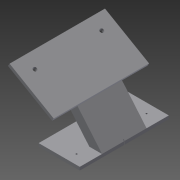
# Autodesk Inventor part: Problem Solving
Saved by Autodesk Inventor 2013 SP1 (Build 170176100, 176)
## iProperties
Created: 2013-04-06
Part Number: Problem Solving
Material: Generic
Document SubType Name: Modeling
Designer: tyler.camp
Density: 1 g/cm^3
Author: tyler.camp
Autodesk Inventor part; units mm, degrees
ref_plane "YZ Plane" through (0, 0, 0) normal (1, 0, 0) x (0, 1, 0)
ref_plane "XZ Plane" through (0, 0, 0) normal (0, 1, 0) x (-1, 0, 0)
ref_plane "XY Plane" through (0, 0, 0) normal (0, 0, 1) x (1, 0, 0)
sketch "Sketch1" plane through (0, 0, 0) normal (0, 0, 1) x (1, 0, 0)
  line L0 (28.2901, 18.0136) -> (77.2705, -40.359)
  line L1 (77.2705, -40.359) -> (51.8705, -40.359)
  line L2 (51.8705, -40.359) -> (-20.9781, 46.4586)
  line L3 (-20.9781, 46.4586) -> (28.2901, 18.0136)
  point P0 (0, 0)
  point P1 (3.656, 32.2361)
  dimension "d0" = 76.2
  dimension "d2" = 25.4
  dimension "d34" = 130
  dimension "d35" = 160
  constraints: 8 end point, 1 horizontal, 1 midpoint, 1 parallel
  measures "d0" distance of L0.start L0.end
  measures "d2" distance of L0.end L1.end
  measures "d34" angle of L1 L2
  measures "d35" angle of L0 L3
extrude "Extrusion1" add sketch "Sketch1" along normal blind 88.9
sketch "Sketch2" plane through (-20.9781, 46.4586, 0) normal (0.5, 0.8660254, 0) x (0, 0, 1)
  line L0 (0, 0) -> (0, 56.89) projected
  line L1 (-50.8, 56.89) -> (139.7, 56.89)
  line L2 (139.7, 56.89) -> (139.7, -44.71)
  line L3 (139.7, -44.71) -> (-50.8, -44.71)
  line L4 (-50.8, -44.71) -> (-50.8, 56.89)
  line L5 (0, 56.89) -> (88.9, 56.89) projected
  point P0 (0, 41.3969)
  point P1 (44.45, 19.4575)
  dimension "d6" = 190.5
  dimension "d8" = 95.25
  dimension "d9" = 101.6
  dimension "d10" = 44.45
  dimension "d11" = 88.9
  dimension "d12" = 56.89
  dimension "d45" = 0
  constraints: 8 end point, 2 parallel, 1 horizontal, 1 perpendicular
  measures "d6" distance of L1.start L1.end
  measures "d8" distance from line of L2 point (44.45, 19.458)
  measures "d9" distance of L1.end L2.end
  measures "d10" distance from line of L0 point (44.45, 19.458)
  measures "d11" distance of L0.end L5.end
  measures "d12" distance of L0.start L0.end
  measures "d45" distance between parallel lines of L5 L1
extrude "Extrusion2" add sketch "Sketch2" along normal blind 6.35
sketch "Sketch3" plane through (-17.8031, 51.9578, 0) normal (0.5, 0.8660254, 0) x (0, 0, 1)
  line L0 (139.7, 56.89) -> (-50.8, 56.89) projected
  circle A0 centre (-22.225, -19.05) radius 3.81
  circle A1 centre (111.125, -19.05) radius 3.81
  line L1 (-50.8, -44.71) -> (139.7, -44.71) projected
  line L2 (44.45, -44.71) -> (44.45, 56.89)
  line L3 (0, 0) -> (88.9, 0) projected
  point P0 (0, 41.3969)
  dimension "d17" = 7.62
  dimension "d18" = 7.62
  dimension "d19" = 0
  dimension "d46" = 133.35
  dimension "d47" = 66.675
  dimension "d86" = 19.05
  constraints: 2 centre point, 2 end point, 2 midpoint
  measures "d17" diameter of A0
  measures "d18" diameter of A1
  measures "d19" vertical distance of A1.centre A0.centre
  measures "d46" distance of A1.centre A0.centre
  measures "d47" distance from line of L2 A0.centre
  measures "d86" distance from line of A0.centre L3
extrude "Extrusion3" cut sketch "Sketch3" against normal up to next
sketch "Sketch6" plane through (-17.8031, 51.9578, 0) normal (0.5, 0.8660254, 0) x (0.8660254, -0.5, 0)
  circle A0 centre (-19.05, 22.225) radius 3.81 projected
  circle A1 centre (-19.05, -111.125) radius 3.81 projected
  line L0 (6.35, 34.925) -> (-44.45, 34.925)
  line L1 (-44.45, 34.925) -> (-44.45, -15.875)
  line L2 (-44.45, -15.875) -> (6.35, -15.875)
  line L3 (6.35, -15.875) -> (6.35, 34.925)
  line L4 (6.35, -73.025) -> (-44.45, -73.025)
  line L5 (-44.45, -73.025) -> (-44.45, -123.825)
  line L6 (-44.45, -123.825) -> (6.35, -123.825)
  line L7 (6.35, -123.825) -> (6.35, -73.025)
  point P0 (41.3969, 0)
  dimension "d52" = 50.8
  dimension "d60" = 25.4
  dimension "d61" = 25.4
  dimension "d62" = 50.8
  dimension "d63" = 12.7
  dimension "d64" = 12.7
  constraints: 16 end point, 4 parallel, 2 equal length, 2 horizontal, 2 perpendicular
  measures "d52" distance of L2.end L0.start
  measures "d60" distance from line of A0.centre L1
  measures "d61" distance from line of A1.centre L5
  measures "d62" distance of L1.end L2.end
  measures "d63" distance from line of L0 A0.centre
  measures "d64" distance from line of L6 A1.centre
extrude "Extrusion5" [suppressed]
sketch "Sketch7" plane through (-18.1206, 51.4079, 0) normal (0.5, 0.8660254, 0) x (0.8660254, -0.5, 0)
  line L0 (6.35, 38.1) -> (-44.45, 38.1) projected
  line L1 (6.35, -76.2) -> (-44.45, -76.2) projected
  line L2 (-44.45, -76.2) -> (-44.45, -127) projected
  line L3 (-44.45, -127) -> (6.35, -127) projected
  line L4 (6.35, -127) -> (6.35, -76.2) projected
  line L5 (-44.45, -12.7) -> (-39.2324, -12.7)
  line L6 (-39.2324, -12.7) -> (-39.2324, 38.1)
  line L7 (-39.2324, 38.1) -> (-44.45, 38.1)
  line L8 (-44.45, 38.1) -> (-44.45, -12.7)
  line L9 (-44.45, -127) -> (-39.2324, -127)
  line L10 (-39.2324, -127) -> (-39.2324, -76.2)
  line L11 (-39.2324, -76.2) -> (-44.45, -76.2)
  line L12 (-44.45, -76.2) -> (-44.45, -127)
  point P0 (41.3969, 0)
  dimension "d56" = 5.2176
  dimension "d57" = 5.2176
  constraints: 16 end point, 4 parallel, 2 horizontal, 2 perpendicular, 2 point on line
  measures "d56" distance between parallel lines of L8 L6
  measures "d57" distance between parallel lines of L10 L2
extrude "Extrusion6" [suppressed]
sketch "Sketch13" plane through (-57.8855, 71.4332, -38.1) normal (-0.8660254, 0.5, 0) x (0, 0, 1)
  line L0 (0, 0) -> (0, 2.54) projected
  circle A0 centre (25.4, 39.096) radius 3.175
  circle A1 centre (139.7, 39.096) radius 3.175
  line L1 (114.3, 0) -> (114.3, 2.54) projected
  point P0 (50.8, 53.34)
  point P1 (0, 53.34)
  point P2 (38.1, -32.9202)
  point P3 (114.3, 53.34)
  dimension "d98" = 6.35
  dimension "d99" = 0
  dimension "d100" = 25.4
  dimension "d101" = 50.8
  dimension "d102" = 25.4
  constraints: 2 centre point, 1 equal radius
  measures "d98" diameter of A0
  measures "d99" vertical distance of A1.centre A0.centre
  measures "d100" distance from line of L0 A0.centre
  measures "d101" distance of point (0, 53.34) point (50.8, 53.34)
  measures "d102" distance from line of L1 A1.centre
extrude "Extrusion11" [suppressed]
sketch "Sketch14" plane through (-57.8855, 71.4332, -38.1) normal (-0.8660254, 0.5, 0) x (0, 0, 1)
  circle A0 centre (25.4, 39.096) radius 3.175 projected
  line L0 (-107.95, 213.721) -> (273.05, 213.721)
  line L1 (273.05, 213.721) -> (273.05, -14.879)
  line L2 (273.05, -14.879) -> (-107.95, -14.879)
  line L3 (-107.95, -14.879) -> (-107.95, 213.721)
  point P0 (38.1, -32.9202)
  dimension "d107" = 381
  dimension "d109" = 228.6
  dimension "d110" = 133.35
  dimension "d111" = 53.975
  constraints: 8 end point, 2 parallel, 1 horizontal, 1 perpendicular
  measures "d107" distance of L0.start L0.end
  measures "d109" distance of L2.end L0.start
  measures "d110" distance from line of A0.centre L3
  measures "d111" distance from line of L2 A0.centre
extrude "Extrusion12" [suppressed]
sketch "Sketch18" plane through (-57.8855, 71.4332, -38.1) normal (0.8660254, -0.5, 0) x (0, 0, -1)
  line L0 (-273.05, -14.879) -> (107.95, -14.879) projected
  line L1 (-273.05, 213.721) -> (-195.9898, 213.721)
  line L2 (-195.9898, 213.721) -> (-195.9898, -14.879)
  line L3 (-195.9898, -14.879) -> (-273.05, -14.879)
  line L4 (-273.05, -14.879) -> (-273.05, 213.721)
  line L5 (107.95, 213.721) -> (30.8898, 213.721)
  line L6 (30.8898, 213.721) -> (30.8898, -14.879)
  line L7 (30.8898, -14.879) -> (107.95, -14.879)
  line L8 (107.95, -14.879) -> (107.95, 213.721)
  point P0 (-38.1, -32.9202)
  constraints: 16 end point, 4 parallel, 2 horizontal, 2 perpendicular, 2 point on line, 1 collinear
extrude "Extrusion14" [suppressed]
sketch "Sketch15" plane through (0, 0, 0) normal (0, 0, 1) x (1, 0, 0)
  line L0 (15.9795, 275.571) -> (4.9809, 281.921) projected
  line L1 (-109.3191, 83.9476) -> (4.9809, 281.921) projected
  line L2 (-98.3205, 77.5976) -> (-109.3191, 83.9476) projected
  line L3 (77.2705, -40.359) -> (28.2901, 18.0136) projected
  line L4 (28.2901, 18.0136) -> (-20.9781, 46.4586) projected
  line L5 (-20.9781, 46.4586) -> (51.8705, -40.359) projected
  line L6 (51.8705, -40.359) -> (77.2705, -40.359) projected
  line L7 (77.2705, -40.359) -> (-405.3295, -40.359)
  line L8 (77.2705, -40.359) -> (204.2705, -40.359)
  line L9 (-98.3205, 77.5976) -> (15.9795, 275.571) projected
  point P0 (0, 0)
  point P1 (-65.325, 58.5476)
  point P2 (48.975, 256.521)
  dimension "d125" = 127
  dimension "d127" = 482.6
  constraints: 4 end point, 3 coincident, 2 collinear
  measures "d125" distance of L7.start L8.end
  measures "d127" distance of L7.start L7.end
sketch "Sketch16" plane through (0, 0, 0) normal (0, 0, 1) x (1, 0, 0)
  line L0 (77.2705, -40.359) -> (-405.3295, -40.359) projected
  line L1 (15.9795, 275.571) -> (4.9809, 281.921) projected
  line L2 (-109.3191, 83.9476) -> (4.9809, 281.921) projected
  line L3 (-98.3205, 77.5976) -> (-109.3191, 83.9476) projected
  line L4 (77.2705, -40.359) -> (204.2705, -40.359) projected
  line L5 (-98.3205, 77.5976) -> (15.9795, 275.571) projected
  point P0 (0, 0)
  point P1 (-65.325, 58.5476)
  point P2 (51.8705, -40.359)
  point P3 (51.8705, -40.359)
  dimension "d129" = 457.2
  dimension "d130" = 322.28
  dimension "d131" = 98.9066
  dimension "d150" = 188.291
  measures "d129" distance of L0.end point (51.87, -40.359)
  measures "d130" distance from line of L4 point (4.981, 281.921)
  measures "d131" distance from line of L0 point (-65.325, 58.548)
  measures "d150" horizontal distance of L4.end L1.start
sketch "Sketch17" plane through (0, 0, 0) normal (0, 0, 1) x (1, 0, 0)
  line L0 (77.2705, -40.359) -> (-405.3295, -40.359) projected
  line L1 (-144.0325, 61.241) -> (-144.0325, -40.359)
  line L2 (-144.0325, -40.359) -> (-42.4325, -40.359)
  line L3 (-42.4325, -40.359) -> (-42.4325, 35.841)
  line L4 (-42.4325, 35.841) -> (-144.0325, 61.241)
  line L5 (77.2705, -40.359) -> (204.2705, -40.359) projected
  point P0 (0, 0)
  point P1 (-93.2325, -40.359)
  dimension "d141" = 101.6
  dimension "d142" = 101.6
  dimension "d146" = 76.2
  dimension "d147" = 297.503
  dimension "d151" = 312.097
  constraints: 8 end point, 2 perpendicular, 1 collinear, 1 midpoint, 1 parallel
  measures "d141" distance of L1.start L1.end
  measures "d142" distance of L1.end L2.end
  measures "d146" distance of L2.end L3.end
  measures "d147" distance of L5.end point (-93.233, -40.359)
  measures "d151" distance of point (-93.233, -40.359) L0.end
extrude "Extrusion13" [suppressed]
sketch "Sketch19" plane through (51.8705, -40.359, 0) normal (0, -1, 0) x (1, 0, 0)
  line L0 (25.4, 0) -> (0, 0) projected
  line L1 (25.4, 0) -> (25.4, 88.9) projected
  line L2 (0, 88.9) -> (25.4, 88.9) projected
  line L3 (0, 0) -> (0, 88.9) projected
  line L4 (25.4, 88.9) -> (25.4, 133.35)
  line L5 (25.4, 133.35) -> (-56.7156, 133.35)
  line L6 (-56.7156, 133.35) -> (-56.7156, 71.7364)
  line L7 (25.4, 0) -> (25.4, -44.45)
  line L8 (25.4, -44.45) -> (-56.7156, -44.45)
  line L9 (-56.7156, -44.45) -> (-56.7156, 17.1636)
  line L10 (-56.7156, 71.7364) -> (-56.7156, 17.1636)
  point P0 (-51.8705, 0)
  dimension "d153" = 90
  dimension "d155" = 90
  dimension "d156" = 90
  dimension "d159" = 90
  dimension "d160" = 44.45
  constraints: 14 end point, 3 equal length, 2 perpendicular
  measures "d153" angle of L0 L7
  measures "d155" angle of L5 L6
  measures "d156" angle of L8 L9
  measures "d159" angle of L4 L2
  measures "d160" distance of L1.end L4.end
extrude "Extrusion15" add sketch "Sketch19" along normal blind 6.35
sketch "Sketch20" plane through (51.8705, -40.359, 0) normal (0, 1, 0) x (1, 0, 0)
  line L0 (25.4, 44.45) -> (25.4, 0) projected
  line L1 (-56.7156, 44.45) -> (25.4, 44.45) projected
  line L2 (25.4, -133.35) -> (-56.7156, -133.35) projected
  line L3 (25.4, -88.9) -> (25.4, -133.35) projected
  circle A0 centre (0, 25.4) radius 1.5875
  circle A1 centre (0, -114.3) radius 1.5875
  point P0 (-51.8705, 0)
  dimension "d161" = 3.175
  dimension "d162" = 19.05
  dimension "d163" = 25.4
  dimension "d164" = 19.05
  dimension "d165" = 25.4
  constraints: 2 centre point, 1 equal radius
  measures "d161" diameter of A0
  measures "d162" distance from line of L1 A0.centre
  measures "d163" distance from line of L0 A0.centre
  measures "d164" distance from line of L2 A1.centre
  measures "d165" distance from line of L3 A1.centre
extrude "Extrusion16" cut sketch "Sketch20" against normal blind 6.35
sketch "Sketch21" plane through (51.8705, -46.709, 0) normal (0, -1, 0) x (1, 0, 0)
  line L0 (25.4, 133.35) -> (-56.7156, 133.35) projected
  line L1 (-56.7156, -44.45) -> (25.4, -44.45) projected
  line L2 (23.5667, 45.085) -> (31.1867, 45.085)
  line L3 (31.1867, 45.085) -> (31.1867, 43.815)
  line L4 (31.1867, 43.815) -> (23.5667, 43.815)
  line L5 (23.5667, 43.815) -> (23.5667, 45.085)
  point P0 (-51.8705, 0)
  dimension "d168" = 1.27
  dimension "d170" = 177.8
  dimension "d171" = 88.265
  dimension "d172" = 7.62
  constraints: 8 end point, 2 parallel, 1 horizontal, 1 perpendicular
  measures "d168" distance of L2.end L3.end
  measures "d170" distance between parallel lines of L1 L0
  measures "d171" distance between parallel lines of L0 L2
  measures "d172" distance of L3.end L4.end
extrude "Extrusion17" cut sketch "Sketch21" against normal blind 25.4
equation "\"d8\" = 0.5 * d6"
equation "\"d10\" = 0.5 * d11"
equation "\"d18\" = d17"
equation "\"d47\" = 0.5 * d46"
equation "\"d61\" = d60"
equation "\"d64\" = d63"
equation "\"d57\" = d56"
equation "\"d100\" = 0.5 * d101"
equation "\"d102\" = d100"
equation "\"d156\" = d155"
equation "\"d164\" = d162"
equation "\"d165\" = d163"
equation "\"d171\" = 0.5 * d170 - 0.5 * d168"
body "Solid1"
